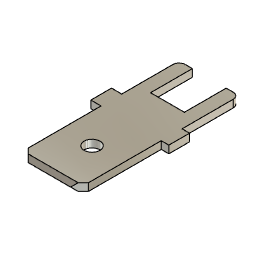
PCB-MALE-TAB v1 (Autodesk Fusion 360 design; units mm, degrees)
Autodesk Fusion 360 part; units mm, degrees
sketch "Sketch1" plane through (0, 0, 0) normal (0, 0, 1) x (1, 0, 0)
  line L0 (-5.9121, -6.5948) -> (-5.9121, 1.1486)
  line L1 (-5.9121, 1.1486) -> (-7, 1.1486)
  line L2 (-7, 1.1486) -> (-7, 3.3486)
  line L3 (-7, 3.3486) -> (-5.9137, 3.3486)
  line L4 (-5.9137, 3.3486) -> (-5.9137, 8.7986)
  line L5 (-5.2637, 9.4486) -> (-4.5, 9.4486)
  line L6 (-4.5, 9.4486) -> (-4.5, 5)
  line L7 (-4.5, 5) -> (-0.9, 5)
  line L8 (-0.9, 5) -> (-0.9, 9.4486)
  line L9 (-0.9, 9.4486) -> (-0.15, 9.4486)
  line L10 (0.5, 8.7986) -> (0.5, 3.3486)
  line L11 (0.5, 3.3486) -> (1.3, 3.3486)
  line L12 (1.3, 3.3486) -> (1.3, 1.1486)
  line L13 (1.3, 1.1486) -> (0.4879, 1.1486)
  line L14 (0.4879, 1.1486) -> (0.4879, -6.5)
  line L15 (0.4879, -6.5) -> (0.4879, -6.5948)
  line L16 (-0.4621, -7.5448) -> (-4.9621, -7.5448)
  line L17 (-5.9121, -6.5948) -> (-4.9621, -7.5448)
  line L18 (-0.4621, -7.5448) -> (0.4879, -6.5948)
  circle A0 centre (-2.7253, -2.9948) radius 0.85
  arc A1 (-5.2637, 9.4486) -> (-5.9137, 8.7986) centre (-5.2637, 8.7986) ccw
  arc A2 (0.5, 8.7986) -> (-0.15, 9.4486) centre (-0.15, 8.7986) ccw
  line L19 (-5.9121, -6.5948) -> (0.4879, -6.5948)
  dimension "d1" = 3.6
  dimension "d2" = 8.3
  dimension "d3" = 6.1
  dimension "d5" = 6.4
  dimension "d6" = 2.2
  dimension "d7" = 4.5
  dimension "d8" = 1.7
  dimension "d9" = 4.55
  dimension "d10" = 0.65
  dimension "d11" = 0.65
  constraint vertical L0
  constraint perpendicular L0 L1
  constraint perpendicular L1 L2
  constraint perpendicular L2 L3
  constraint perpendicular L3 L4
  constraint perpendicular L4 L5
  constraint perpendicular L3 L6
  constraint perpendicular L6 L7
  constraint perpendicular L3 L8
  constraint perpendicular L6 L9
  constraint perpendicular L3 L10
  constraint perpendicular L4 L11
  constraint perpendicular L1 L12
  constraint perpendicular L12 L13
  constraint perpendicular L1 L14
  constraint parallel L14 L15
  constraint equal L2 L12
  constraint perpendicular L17 L18
  constraint coincident L18 L16.start
  constraint horizontal L16
  constraint tangent L5 A1
  constraint tangent L4 A1
  constraint tangent L9 A2
  constraint tangent L10 A2
  constraint equal L17 L18
  constraint coincident L16.start L18.start
  constraint horizontal L19
  measures "d1" distance of L6.end L7.end
  measures "d2" distance of L2.end L11.end
  measures "d3" distance of L3.end L5
  measures "d5" horizontal distance of L0.start L14.end
  measures "d6" distance of L11.end L12.end
  measures "d7" horizontal distance of L16.end L16.start
  measures "d8" diameter of A0
  measures "d9" distance of L16 A0.centre
  measures "d10" radius of A1
  measures "d11" radius of A2
extrude "Extrude1" add sketch "Sketch1" along normal blind 0.8
chamfer "Chamfer1" distance 0.4 angle 45 2 edges at (-2.7121, -7.5448, 0.8) (-2.7121, -7.5448, 0)
